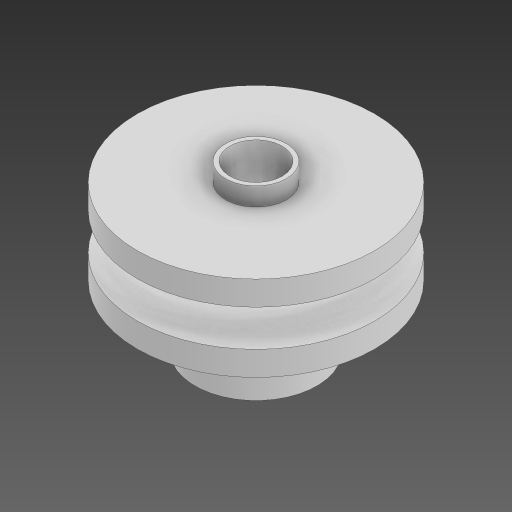
# Autodesk Inventor part: koleso_left
Saved by Autodesk Inventor 2023 (Build 270158000, 158)
## iProperties
Created: 2025-05-29
Part Number: koleso_left
Material: Типовые
Document SubType Name: Modeling
Designer: daa
Density: 1 g/cm^3
Appearance: По умолчанию
Author: daa
Autodesk Inventor part; units mm, degrees
ref_plane "YZ Plane" through (0, 0, 0) normal (1, 0, 0) x (0, 1, 0)
ref_plane "XZ Plane" through (0, 0, 0) normal (0, 1, 0) x (-1, 0, 0)
ref_plane "XY Plane" through (0, 0, 0) normal (0, 0, 1) x (1, 0, 0)
sketch "Эскиз1" plane through (0, 0, 0) normal (0, 1, 0) x (-1, 0, 0)
  circle A0 centre (0, 0) radius 9.75
  dimension "d0" = 19.5
  constraints: 1 centre point, 1 coincident
  measures "d0" diameter of A0
extrude "Выдавливание1" add sketch "Эскиз1" along normal blind 2
sketch "Эскиз5" plane through (0, 0, 0) normal (0, -1, 0) x (1, 0, 0)
  line L0 (5, -5) -> (-5, -5)
  line L1 (-5, -5) -> (-5, 5)
  line L2 (-5, 5) -> (5, 5)
  line L3 (5, 5) -> (5, -5)
  point P0 (0, 0)
  dimension "d12" = 10
  dimension "d13" = 10
  dimension "d17" = 5
  dimension "d27" = 5
  constraints: 8 end point, 2 parallel, 1 horizontal, 1 perpendicular
  measures "d12" distance of L1.end L2.end
  measures "d13" distance of L0.end L1.end
  measures "d17" distance from line of point (0, 0) L3
  measures "d27" horizontal distance of L0.end point (0, 0)
extrude "Выдавливание5" add sketch "Эскиз5" along normal blind 5
sketch "Эскиз6" plane through (-5, 0, -5) normal (-1, 0, 0) x (0, 0, 1)
  circle A0 centre (5, -2.5) radius 1.35
  line L0 (10, -5) -> (0, -5) projected
  line L1 (0, 0) -> (0, -5) projected
  point P0 (5, 0)
  point P1 (0, -2.5)
  dimension "d30" = 2.7
  dimension "d31" = 2.5
  dimension "d32" = 5
  constraints: 1 centre point, 1 midpoint
  measures "d30" diameter of A0
  measures "d31" distance from line of L0 A0.centre
  measures "d32" distance of point (0, -2.5) A0.centre
extrude "Выдавливание6" cut sketch "Эскиз6" against normal blind 15.75
fillet "Сопряжение1" radius 5 4 edges at (5, -2.5, 5) (-5, -2.5, 5) (-5, -2.5, -5) (5, -2.5, -5)
sketch "Эскиз11" plane through (0, 2, 0) normal (0, 1, 0) x (1, 0, 0)
  circle A0 centre (0, 0) radius 5
  dimension "d47" = 10
  constraints: 1 centre point, 1 coincident
  measures "d47" diameter of A0
extrude "Выдавливание9" add sketch "Эскиз11" along normal blind 3
sketch "Эскиз12" plane through (0, 5, 0) normal (0, 1, 0) x (1, 0, 0)
  circle A0 centre (0, 0) radius 9.75
  dimension "d50" = 19.5
  constraints: 1 centre point, 1 coincident
  measures "d50" diameter of A0
extrude "Выдавливание10" add sketch "Эскиз12" along normal blind 2
sketch "Эскиз14" plane through (0, 7, 0) normal (0, 1, 0) x (1, 0, 0)
  circle A0 centre (0, 0) radius 2.5
  dimension "d56" = 5
  constraints: 1 centre point, 1 coincident
  measures "d56" diameter of A0
extrude "Выдавливание12" add sketch "Эскиз14" along normal blind 1.5
sketch "Эскиз15" plane through (0, 8.5, 0) normal (0, 1, 0) x (1, 0, 0)
  circle A0 centre (0, 0) radius 2.15
  dimension "d59" = 4.3
  constraints: 1 centre point, 1 coincident
  measures "d59" diameter of A0
extrude "Выдавливание13" cut sketch "Эскиз15" against normal blind 33.5
